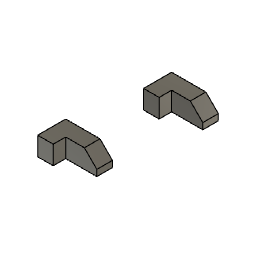
Drawing Projections (Autodesk Fusion 360 design; units mm, degrees)
Autodesk Fusion 360 part; units mm, degrees
sketch "Sketch1" plane through (0, 0, 0) normal (0, 0, 1) x (1, 0, 0)
  line L0 (-25, -20) -> (-25, 25)
  line L1 (-25, 25) -> (50, 25)
  line L2 (50, 25) -> (50, 0)
  line L3 (50, 0) -> (0, 0)
  line L4 (0, 0) -> (0, -20)
  line L5 (0, -20) -> (-25, -20)
  dimension "d1" = 25
  dimension "d2" = 25
  dimension "d3" = 75
  dimension "d4" = 45
  constraint vertical L0
  constraint perpendicular L0 L1
  constraint perpendicular L1 L2
  constraint coincident L3.end L4.start
  constraint perpendicular L3 L4
  constraint horizontal L3
  constraint horizontal L5
  measures "d1" distance of L0.start L4.end
  measures "d2" distance of L1.end L2.end
  measures "d3" distance of L0.end L1.end
  measures "d4" distance of L0.start L0.end
extrude "Extrude1" add sketch "Sketch1" along normal blind 30 makes body 1
chamfer "Chamfer1" distance 20 angle 45 1 edges at (50, 12.5, 30) on bodies 1
move_body "Move1" bodies 1 to x (1, 0, 0) y (0, 1, 0) z (0, 0, 1) at (80, 0, 70)
copy_body "CopyPasteBodies1" bodies 1 makes body 2
move_body "Move2" bodies 2 to x (1, 0, 0) y (0, 1, 0) z (0, 0, 1) at (-170, 0, -150)
sketch "Right" plane through (0, 0, 0) normal (1, 0, 0) x (0, 1, 0)
  line L0 (75, 150) -> (-75, 150)
  line L1 (-75, 150) -> (-75, -150)
  line L2 (-75, -150) -> (75, -150)
  line L3 (75, -150) -> (75, 150)
  line L4 (-75, 0) -> (75, 0)
  line L5 (25, 100) -> (-20, 100)
  line L6 (25, 70) -> (25, 100)
  line L7 (-20, 70) -> (-20, 100)
  line L8 (-20, 70) -> (25, 70)
  line L9 (25, -50) -> (-20, -50)
  line L10 (25, -80) -> (25, -50)
  line L11 (-20, -80) -> (-20, -50)
  line L12 (-20, -80) -> (25, -80)
  line L13 (0, 70) -> (0, 100)
  line L14 (0, 80) -> (25, 80)
  line L15 (0, -80) -> (0, -50)
  line L16 (0, -70) -> (25, -70)
  dimension "d8" = 150
  dimension "d9" = 300
  constraint horizontal L0
  constraint perpendicular L0 L1
  constraint parallel L0 L2
  constraint parallel L1 L3
  constraint midpoint L1 L4.start
  constraint midpoint L3 L4.end
  measures "d8" distance of L1.end L2.end
  measures "d9" distance of L0.end L1.end
sketch "Top" plane through (0, 0, 0) normal (0, 0, 1) x (1, 0, 0)
  line L0 (150, -75) -> (-150, -75)
  line L1 (-150, -75) -> (-150, 75)
  line L2 (-150, 75) -> (150, 75)
  line L3 (150, 75) -> (150, -75)
  line L4 (0, -75) -> (0, 75)
  line L5 (110, 0) -> (110, 25)
  line L6 (110, 25) -> (55, 25)
  line L7 (55, 25) -> (55, -20)
  line L8 (55, -20) -> (80, -20)
  line L9 (80, -20) -> (80, 0)
  line L10 (80, 0) -> (110, 0)
  line L11 (130, 25) -> (110, 25)
  line L12 (110, 25) -> (110, 0)
  line L13 (110, 0) -> (130, 0)
  line L14 (130, 0) -> (130, 25)
  line L15 (-60, 0) -> (-60, 25)
  line L16 (-60, 25) -> (-115, 25)
  line L17 (-115, 25) -> (-115, -20)
  line L18 (-115, -20) -> (-90, -20)
  line L19 (-90, -20) -> (-90, 0)
  line L20 (-90, 0) -> (-60, 0)
  line L21 (-40, 25) -> (-60, 25)
  line L22 (-60, 25) -> (-60, 0)
  line L23 (-60, 0) -> (-40, 0)
  line L24 (-40, 0) -> (-40, 25)
  dimension "d10" = 300
  dimension "d11" = 150
  constraint horizontal L0
  constraint perpendicular L0 L1
  constraint parallel L0 L2
  constraint parallel L1 L3
  constraint midpoint L0 L4.start
  constraint midpoint L2 L4.end
  measures "d10" distance of L1.end L2.end
  measures "d11" distance of L0.end L1.end
sketch "Sketch4" plane through (0, 0, 0) normal (0, 0, 1) x (1, 0, 0)
  line L0 (20, 60) -> (165, 60)
  line L1 (165, 60) -> (165, -55)
  line L2 (165, -55) -> (20, -55)
  line L3 (20, -55) -> (20, 60)
  line L4 (-150, 60) -> (-5, 60)
  line L5 (-5, 60) -> (-5, -55)
  line L6 (-5, -55) -> (-150, -55)
  line L7 (-150, -55) -> (-150, 60)
  line L8 (130, 0) -> (130, 25)
  line L9 (55, 25) -> (55, -20)
  line L10 (-40, 0) -> (-40, 25)
  line L11 (-60, 25) -> (-115, 25)
  line L12 (-115, -20) -> (-90, -20)
  dimension "d12" = 35
  dimension "d13" = 35
  dimension "d14" = 35
  dimension "d15" = 35
  dimension "d16" = 35
  constraint horizontal L0
  constraint vertical L1
  constraint horizontal L2
  constraint vertical L3
  constraint horizontal L4
  constraint vertical L5
  constraint horizontal L6
  constraint vertical L7
  constraint equal L3 L5
  constraint equal L0 L4
  constraint collinear L0 L4
  measures "d12" distance of L1 L8
  measures "d13" distance of L3 L9
  measures "d14" distance of L5 L10
  measures "d15" distance of L4 L11
  measures "d16" distance of L6 L12
extrude "Extrude2" add sketch "Sketch4" along normal blind 75 from surface at 50 separate body contours L0 L1 L2 L3 makes body 3
extrude "Extrude3" add sketch "Sketch4" against normal blind 75 from surface at -25 separate body contours L4 L5 L6 L7 makes body 4
sketch "1st Front" plane through (0, 60, 0) normal (0, 1, 0) x (-1, 0, 0)
  line L0 (-165, 50) -> (-20, 50)
  line L1 (-20, 50) -> (-20, 125)
  line L2 (-20, 125) -> (-165, 125)
  line L3 (-165, 125) -> (-165, 50)
  line L4 (-110, 100) -> (-130, 80)
  line L5 (-130, 80) -> (-130, 70)
  line L6 (-130, 70) -> (-55, 70)
  line L7 (-55, 70) -> (-55, 100)
  line L8 (-55, 100) -> (-110, 100)
  line L9 (-80, 70) -> (-80, 100)
sketch "1st Top" plane through (0, 0, 50) normal (0, 0, -1) x (1, 0, 0)
  line L0 (165, 55) -> (20, 55)
  line L1 (20, 55) -> (20, -60)
  line L2 (20, -60) -> (165, -60)
  line L3 (165, -60) -> (165, 55)
  line L4 (110, 0) -> (110, -25)
  line L5 (110, -25) -> (55, -25)
  line L6 (55, -25) -> (55, 20)
  line L7 (55, 20) -> (80, 20)
  line L8 (80, 20) -> (80, 0)
  line L9 (80, 0) -> (110, 0)
  line L10 (130, -25) -> (110, -25)
  line L11 (110, -25) -> (110, 0)
  line L12 (110, 0) -> (130, 0)
  line L13 (130, 0) -> (130, -25)
sketch "1st Right" plane through (20, 0, 0) normal (-1, 0, 0) x (0, -1, 0)
  line L0 (-60, 50) -> (55, 50)
  line L1 (55, 50) -> (55, 125)
  line L2 (55, 125) -> (-60, 125)
  line L3 (-60, 125) -> (-60, 50)
  line L4 (20, 70) -> (0, 70)
  line L5 (0, 70) -> (0, 100)
  line L6 (0, 100) -> (20, 100)
  line L7 (20, 100) -> (20, 70)
  line L8 (-25, 80) -> (-25, 100)
  line L9 (-25, 100) -> (0, 100)
  line L10 (0, 100) -> (0, 80)
  line L11 (0, 80) -> (-25, 80)
  line L12 (-25, 80) -> (0, 80)
  line L13 (0, 80) -> (0, 70)
  line L14 (0, 70) -> (-25, 70)
  line L15 (-25, 70) -> (-25, 80)
sketch "3rd Top" plane through (0, 0, -25) normal (0, 0, 1) x (-1, 0, 0)
  line L0 (150, 55) -> (5, 55)
  line L1 (5, 55) -> (5, -60)
  line L2 (5, -60) -> (150, -60)
  line L3 (150, -60) -> (150, 55)
  line L4 (60, 0) -> (60, -25)
  line L5 (60, -25) -> (115, -25)
  line L6 (115, -25) -> (115, 20)
  line L7 (115, 20) -> (90, 20)
  line L8 (90, 20) -> (90, 0)
  line L9 (90, 0) -> (60, 0)
  line L10 (40, -25) -> (60, -25)
  line L11 (60, -25) -> (60, 0)
  line L12 (60, 0) -> (40, 0)
  line L13 (40, 0) -> (40, -25)
sketch "3rd Right" plane through (-5, 0, 0) normal (1, 0, 0) x (0, 1, 0)
  line L0 (60, -25) -> (-55, -25)
  line L1 (-55, -25) -> (-55, -100)
  line L2 (-55, -100) -> (60, -100)
  line L3 (60, -100) -> (60, -25)
  line L4 (-20, -80) -> (0, -80)
  line L5 (0, -80) -> (0, -50)
  line L6 (0, -50) -> (-20, -50)
  line L7 (-20, -50) -> (-20, -80)
  line L8 (25, -70) -> (25, -50)
  line L9 (25, -50) -> (0, -50)
  line L10 (0, -50) -> (0, -70)
  line L11 (0, -70) -> (25, -70)
  line L12 (25, -70) -> (0, -70)
  line L13 (0, -70) -> (0, -80)
  line L14 (0, -80) -> (25, -80)
  line L15 (25, -80) -> (25, -70)
sketch "3rd Front" plane through (0, -55, 0) normal (0, -1, 0) x (1, 0, 0)
  line L0 (-5, -25) -> (-150, -25)
  line L1 (-150, -25) -> (-150, -100)
  line L2 (-150, -100) -> (-5, -100)
  line L3 (-5, -100) -> (-5, -25)
  line L4 (-115, -80) -> (-90, -80)
  line L5 (-90, -80) -> (-90, -50)
  line L6 (-90, -50) -> (-115, -50)
  line L7 (-115, -50) -> (-115, -80)
  line L8 (-40, -70) -> (-60, -50)
  line L9 (-60, -50) -> (-90, -50)
  line L10 (-90, -50) -> (-90, -80)
  line L11 (-90, -80) -> (-40, -80)
  line L12 (-40, -80) -> (-40, -70)
hidden bodies 3 4
named bodies: "1st Proj", "3rd Proj", "1st Proj Cube", "3rd Proj Cube"
